45 teeth ring (Autodesk Fusion 360 design; units mm, degrees)
description: Spur Gear; Module: 1.27; Num Teeth: 45; Pressure Angle: 20.0; Backlash: 0.00 mm
part number: 2026-06-12-01-57-33-640
Autodesk Fusion 360 part; units mm, degrees
(part 1 of 5)
sketch "Base Circle" plane through (0, 0, 0) normal (0, 0, 1) x (1, 0, 0)
  circle A0 centre (0, 0) radius 27.1056
  circle A1 centre (0, 0) radius 2.5
extrude "Extrude1" add sketch "Base Circle" along normal blind 1 makes body 1
sketch "Gear Tooth" plane through (0, 0, 0) normal (0, 0, 1) x (1, 0, 0)
  spline S0 degree 5 poles (26.8184, -1.337) (26.8271, -1.337) (26.8445, -1.337) (26.8706, -1.3368) (26.9054, -1.3362) (26.9489, -1.3346) (26.9925, -1.3324) (27.036, -1.3295) (27.0796, -1.3259) (27.1232, -1.3218) (27.1667, -1.3171) (27.2103, -1.3119) (27.2539, -1.3063) (27.2974, -1.3003) (27.341, -1.294) (27.3845, -1.2874) (27.4281, -1.2804) (27.4716, -1.273) (27.5152, -1.2653) (27.5587, -1.2573) (27.6022, -1.249) (27.6457, -1.2403) (27.6892, -1.2313) (27.7327, -1.2221) (27.7762, -1.2126) (27.8196, -1.2028) (27.8631, -1.1927) (27.9065, -1.1824) (27.9499, -1.1718) (27.9933, -1.1609) (28.0367, -1.1498) (28.0801, -1.1384) (28.1235, -1.1268) (28.1668, -1.115) (28.2101, -1.1029) (28.2534, -1.0905) (28.2967, -1.0779) (28.34, -1.0651) (28.3833, -1.0521) (28.4265, -1.0389) (28.4697, -1.0254) (28.513, -1.0117) (28.5561, -0.9978) (28.5993, -0.9837) (28.6424, -0.9693) (28.6856, -0.9548) (28.7287, -0.94) (28.7718, -0.925) (28.8148, -0.9099) (28.8579, -0.8945) (28.9009, -0.8789) (28.9439, -0.8631) (28.9868, -0.8471) (29.0298, -0.831) (29.0727, -0.8146) (29.1156, -0.798) (29.1585, -0.7813) (29.2013, -0.7643) (29.2442, -0.7472) (29.287, -0.7299) (29.3298, -0.7124) (29.3725, -0.6947) (29.4152, -0.6768) (29.4579, -0.6588) (29.5006, -0.6405) (29.5433, -0.6221) (29.5859, -0.6035) (29.6285, -0.5847) (29.671, -0.5658) (29.7136, -0.5466) (29.7561, -0.5273) (29.7901, -0.5118) (29.8155, -0.5) (29.8325, -0.4921) (29.841, -0.4882) knots 0 0 0 0 0 0 0.01428571 0.02857143 0.04285714 0.05714286 0.07142857 0.08571429 0.1 0.11428571 0.12857143 0.14285714 0.15714286 0.17142857 0.18571429 0.2 0.21428571 0.22857143 0.24285714 0.25714286 0.27142857 0.28571429 0.3 0.31428571 0.32857143 0.34285714 0.35714286 0.37142857 0.38571429 0.4 0.41428571 0.42857143 0.44285714 0.45714286 0.47142857 0.48571429 0.5 0.51428571 0.52857143 0.54285714 0.55714286 0.57142857 0.58571429 0.6 0.61428571 0.62857143 0.64285714 0.65714286 0.67142857 0.68571429 0.7 0.71428571 0.72857143 0.74285714 0.75714286 0.77142857 0.78571429 0.8 0.81428571 0.82857143 0.84285714 0.85714286 0.87142857 0.88571429 0.9 0.91428571 0.92857143 0.94285714 0.95714286 0.97142857 0.98571429 1 1 1 1 1 1
  spline S1 degree 5 poles (26.8184, 1.337) (26.8271, 1.337) (26.8445, 1.337) (26.8706, 1.3368) (26.9054, 1.3362) (26.9489, 1.3346) (26.9925, 1.3324) (27.036, 1.3295) (27.0796, 1.3259) (27.1232, 1.3218) (27.1667, 1.3171) (27.2103, 1.3119) (27.2539, 1.3063) (27.2974, 1.3003) (27.341, 1.294) (27.3845, 1.2874) (27.4281, 1.2804) (27.4716, 1.273) (27.5152, 1.2653) (27.5587, 1.2573) (27.6022, 1.249) (27.6457, 1.2403) (27.6892, 1.2313) (27.7327, 1.2221) (27.7762, 1.2126) (27.8196, 1.2028) (27.8631, 1.1927) (27.9065, 1.1824) (27.9499, 1.1718) (27.9933, 1.1609) (28.0367, 1.1498) (28.0801, 1.1384) (28.1235, 1.1268) (28.1668, 1.115) (28.2101, 1.1029) (28.2534, 1.0905) (28.2967, 1.0779) (28.34, 1.0651) (28.3833, 1.0521) (28.4265, 1.0389) (28.4697, 1.0254) (28.513, 1.0117) (28.5561, 0.9978) (28.5993, 0.9837) (28.6424, 0.9693) (28.6856, 0.9548) (28.7287, 0.94) (28.7718, 0.925) (28.8148, 0.9099) (28.8579, 0.8945) (28.9009, 0.8789) (28.9439, 0.8631) (28.9868, 0.8471) (29.0298, 0.831) (29.0727, 0.8146) (29.1156, 0.798) (29.1585, 0.7813) (29.2013, 0.7643) (29.2442, 0.7472) (29.287, 0.7299) (29.3298, 0.7124) (29.3725, 0.6947) (29.4152, 0.6768) (29.4579, 0.6588) (29.5006, 0.6405) (29.5433, 0.6221) (29.5859, 0.6035) (29.6285, 0.5847) (29.671, 0.5658) (29.7136, 0.5466) (29.7561, 0.5273) (29.7901, 0.5118) (29.8155, 0.5) (29.8325, 0.4921) (29.841, 0.4882) knots 0 0 0 0 0 0 0.01428571 0.02857143 0.04285714 0.05714286 0.07142857 0.08571429 0.1 0.11428571 0.12857143 0.14285714 0.15714286 0.17142857 0.18571429 0.2 0.21428571 0.22857143 0.24285714 0.25714286 0.27142857 0.28571429 0.3 0.31428571 0.32857143 0.34285714 0.35714286 0.37142857 0.38571429 0.4 0.41428571 0.42857143 0.44285714 0.45714286 0.47142857 0.48571429 0.5 0.51428571 0.52857143 0.54285714 0.55714286 0.57142857 0.58571429 0.6 0.61428571 0.62857143 0.64285714 0.65714286 0.67142857 0.68571429 0.7 0.71428571 0.72857143 0.74285714 0.75714286 0.77142857 0.78571429 0.8 0.81428571 0.82857143 0.84285714 0.85714286 0.87142857 0.88571429 0.9 0.91428571 0.92857143 0.94285714 0.95714286 0.97142857 0.98571429 1 1 1 1 1 1
  arc A0 (29.841, -0.4882) -> (29.841, 0.4882) centre (0, 0) ccw
  line L0 (26.8184, 1.337) -> (26.8184, -1.337)
  point P0 (27.0328, -1.3296)
  point P1 (27.248, -1.307)
  point P2 (27.4636, -1.2743)
  point P3 (27.6795, -1.2333)
  point P4 (27.8956, -1.1849)
  point P5 (28.1119, -1.1299)
  point P6 (28.3282, -1.0686)
  point P7 (28.5446, -1.0015)
  point P8 (28.761, -0.9287)
  point P9 (28.9773, -0.8507)
  point P10 (29.1935, -0.7674)
  point P11 (29.4095, -0.6792)
  point P12 (29.6254, -0.586)
  point P13 (27.0328, 1.3296)
  point P14 (27.248, 1.307)
  point P15 (27.4636, 1.2743)
  point P16 (27.6795, 1.2333)
  point P17 (27.8956, 1.1849)
  point P18 (28.1119, 1.1299)
  point P19 (28.3282, 1.0686)
  point P20 (28.5446, 1.0015)
  point P21 (28.761, 0.9287)
  point P22 (28.9773, 0.8507)
  point P23 (29.1935, 0.7674)
  point P24 (29.4095, 0.6792)
  point P25 (29.6254, 0.586)
extrude "Extrude2" add sketch "Gear Tooth" along normal blind 1 bodies 1
fillet "Fillet1" radius 0.2 2 edges at (27.0731, 1.3263, 0.5) (27.0731, -1.3263, 0.5) on bodies 1
pattern_circular "C-Pattern1" count 45 over 360 about axis through (0, 0, 0) along (0, 0, 1) of "Extrude2", "Fillet1"
sketch "Diametrial Pitch Circle" plane through (0, 0, 0) normal (0, 0, 1) x (1, 0, 0)
  circle A0 centre (0, 0) radius 28.575 construction
sketch "Sketch4" plane through (0, 0, 1) normal (0, 0, 1) x (1, 0, 0)
  arc A0 (27.0091, -2.2856) -> (27.0643, -1.4956) centre (0, 0) ccw
  spline S0 degree 3 poles (27.2384, -1.3082) (27.2125, -1.3116) (27.1876, -1.3199) (27.1423, -1.3457) (27.1225, -1.3629) (27.0939, -1.3995) (27.0839, -1.4173) (27.0696, -1.4553) (27.0654, -1.4753) (27.0643, -1.4956) knots 0 0 0 0 0.007813 0.007813 0.015626 0.015626 0.021719 0.021719 0.027811 0.027811 0.027811 0.027811
  spline S1 degree 5 poles (27.2384, -1.3082) (27.2415, -1.3078) (27.2533, -1.3063) (27.2738, -1.3036) (27.303, -1.2995) (27.341, -1.294) (27.3845, -1.2874) (27.4281, -1.2804) (27.4716, -1.273) (27.5152, -1.2653) (27.5587, -1.2573) (27.6022, -1.249) (27.6457, -1.2403) (27.6892, -1.2313) (27.7327, -1.2221) (27.7762, -1.2126) (27.8196, -1.2028) (27.8631, -1.1927) (27.9065, -1.1824) (27.9499, -1.1718) (27.9933, -1.1609) (28.0367, -1.1498) (28.0801, -1.1384) (28.1235, -1.1268) (28.1668, -1.115) (28.2101, -1.1029) (28.2534, -1.0905) (28.2967, -1.0779) (28.34, -1.0651) (28.3833, -1.0521) (28.4265, -1.0389) (28.4697, -1.0254) (28.513, -1.0117) (28.5561, -0.9978) (28.5993, -0.9837) (28.6424, -0.9693) (28.6856, -0.9548) (28.7287, -0.94) (28.7718, -0.925) (28.8148, -0.9099) (28.8579, -0.8945) (28.9009, -0.8789) (28.9439, -0.8631) (28.9868, -0.8471) (29.0298, -0.831) (29.0727, -0.8146) (29.1156, -0.798) (29.1585, -0.7813) (29.2013, -0.7643) (29.2442, -0.7472) (29.287, -0.7299) (29.3298, -0.7124) (29.3725, -0.6947) (29.4152, -0.6768) (29.4579, -0.6588) (29.5006, -0.6405) (29.5433, -0.6221) (29.5859, -0.6035) (29.6285, -0.5847) (29.671, -0.5658) (29.7136, -0.5466) (29.7561, -0.5273) (29.7901, -0.5118) (29.8155, -0.5) (29.8325, -0.4921) (29.841, -0.4882) knots 0.13777296 0.13777296 0.13777296 0.13777296 0.13777296 0.13777296 0.14285714 0.15714286 0.17142857 0.18571429 0.2 0.21428571 0.22857143 0.24285714 0.25714286 0.27142857 0.28571429 0.3 0.31428571 0.32857143 0.34285714 0.35714286 0.37142857 0.38571429 0.4 0.41428571 0.42857143 0.44285714 0.45714286 0.47142857 0.48571429 0.5 0.51428571 0.52857143 0.54285714 0.55714286 0.57142857 0.58571429 0.6 0.61428571 0.62857143 0.64285714 0.65714286 0.67142857 0.68571429 0.7 0.71428571 0.72857143 0.74285714 0.75714286 0.77142857 0.78571429 0.8 0.81428571 0.82857143 0.84285714 0.85714286 0.87142857 0.88571429 0.9 0.91428571 0.92857143 0.94285714 0.95714286 0.97142857 0.98571429 1 1 1 1 1 1
  arc A1 (29.841, -0.4882) -> (29.841, 0.4882) centre (0, 0) ccw
  spline S2 degree 5 poles (29.841, 0.4882) (29.8325, 0.4921) (29.8155, 0.5) (29.7901, 0.5118) (29.7561, 0.5273) (29.7136, 0.5466) (29.671, 0.5658) (29.6285, 0.5847) (29.5859, 0.6035) (29.5433, 0.6221) (29.5006, 0.6405) (29.4579, 0.6588) (29.4152, 0.6768) (29.3725, 0.6947) (29.3298, 0.7124) (29.287, 0.7299) (29.2442, 0.7472) (29.2013, 0.7643) (29.1585, 0.7813) (29.1156, 0.798) (29.0727, 0.8146) (29.0298, 0.831) (28.9868, 0.8471) (28.9439, 0.8631) (28.9009, 0.8789) (28.8579, 0.8945) (28.8148, 0.9099) (28.7718, 0.925) (28.7287, 0.94) (28.6856, 0.9548) (28.6424, 0.9693) (28.5993, 0.9837) (28.5561, 0.9978) (28.513, 1.0117) (28.4697, 1.0254) (28.4265, 1.0389) (28.3833, 1.0521) (28.34, 1.0651) (28.2967, 1.0779) (28.2534, 1.0905) (28.2101, 1.1029) (28.1668, 1.115) (28.1235, 1.1268) (28.0801, 1.1384) (28.0367, 1.1498) (27.9933, 1.1609) (27.9499, 1.1718) (27.9065, 1.1824) (27.8631, 1.1927) (27.8196, 1.2028) (27.7762, 1.2126) (27.7327, 1.2221) (27.6892, 1.2313) (27.6457, 1.2403) (27.6022, 1.249) (27.5587, 1.2573) (27.5152, 1.2653) (27.4716, 1.273) (27.4281, 1.2804) (27.3845, 1.2874) (27.341, 1.294) (27.303, 1.2995) (27.2738, 1.3036) (27.2533, 1.3063) (27.2415, 1.3078) (27.2384, 1.3082) knots -1 -1 -1 -1 -1 -1 -0.98571429 -0.97142857 -0.95714286 -0.94285714 -0.92857143 -0.91428571 -0.9 -0.88571429 -0.87142857 -0.85714286 -0.84285714 -0.82857143 -0.81428571 -0.8 -0.78571429 -0.77142857 -0.75714286 -0.74285714 -0.72857143 -0.71428571 -0.7 -0.68571429 -0.67142857 -0.65714286 -0.64285714 -0.62857143 -0.61428571 -0.6 -0.58571429 -0.57142857 -0.55714286 -0.54285714 -0.52857143 -0.51428571 -0.5 -0.48571429 -0.47142857 -0.45714286 -0.44285714 -0.42857143 -0.41428571 -0.4 -0.38571429 -0.37142857 -0.35714286 -0.34285714 -0.32857143 -0.31428571 -0.3 -0.28571429 -0.27142857 -0.25714286 -0.24285714 -0.22857143 -0.21428571 -0.2 -0.18571429 -0.17142857 -0.15714286 -0.14285714 -0.13777296 -0.13777296 -0.13777296 -0.13777296 -0.13777296 -0.13777296
  spline S3 degree 3 poles (27.0643, 1.4956) (27.0658, 1.4696) (27.0723, 1.4441) (27.0947, 1.3971) (27.1103, 1.376) (27.1447, 1.3448) (27.1617, 1.3335) (27.1986, 1.3165) (27.2182, 1.3109) (27.2384, 1.3082) knots 0 0 0 0 0.007813 0.007813 0.015626 0.015626 0.021719 0.021719 0.027811 0.027811 0.027811 0.027811
  arc A2 (27.0643, 1.4956) -> (27.0091, 2.2856) centre (0, 0) ccw
  spline S4 degree 3 poles (27.1553, 2.4953) (27.1302, 2.4884) (27.1067, 2.4767) (27.0655, 2.4448) (27.0482, 2.4251) (27.025, 2.3849) (27.0176, 2.3659) (27.0087, 2.3262) (27.0074, 2.3059) (27.0091, 2.2856) knots 0 0 0 0 0.007813 0.007813 0.015626 0.015626 0.021719 0.021719 0.027811 0.027811 0.027811 0.027811
  spline S5 degree 5 poles (27.1553, 2.4953) (27.1584, 2.4962) (27.1698, 2.4993) (27.1898, 2.5049) (27.2182, 2.513) (27.255, 2.5237) (27.2972, 2.5364) (27.3393, 2.5493) (27.3814, 2.5627) (27.4235, 2.5764) (27.4655, 2.5904) (27.5074, 2.6047) (27.5493, 2.6193) (27.5911, 2.6342) (27.6329, 2.6494) (27.6746, 2.6649) (27.7163, 2.6807) (27.7579, 2.6967) (27.7995, 2.713) (27.841, 2.7295) (27.8825, 2.7463) (27.9239, 2.7633) (27.9653, 2.7806) (28.0066, 2.7982) (28.0479, 2.816) (28.0891, 2.834) (28.1303, 2.8522) (28.1714, 2.8707) (28.2125, 2.8894) (28.2535, 2.9083) (28.2945, 2.9275) (28.3354, 2.9468) (28.3763, 2.9664) (28.4171, 2.9862) (28.4579, 3.0062) (28.4986, 3.0264) (28.5393, 3.0468) (28.5799, 3.0674) (28.6205, 3.0882) (28.661, 3.1092) (28.7015, 3.1305) (28.7419, 3.1519) (28.7823, 3.1735) (28.8226, 3.1953) (28.8629, 3.2173) (28.9032, 3.2395) (28.9433, 3.2618) (28.9835, 3.2844) (29.0235, 3.3071) (29.0636, 3.3301) (29.1035, 3.3532) (29.1435, 3.3765) (29.1833, 3.3999) (29.2232, 3.4236) (29.2629, 3.4474) (29.3027, 3.4714) (29.3423, 3.4956) (29.3819, 3.5199) (29.4215, 3.5445) (29.461, 3.5691) (29.5005, 3.594) (29.5399, 3.619) (29.5714, 3.6392) (29.595, 3.6544) (29.6107, 3.6646) (29.6185, 3.6697) knots 0.13777296 0.13777296 0.13777296 0.13777296 0.13777296 0.13777296 0.14285714 0.15714286 0.17142857 0.18571429 0.2 0.21428571 0.22857143 0.24285714 0.25714286 0.27142857 0.28571429 0.3 0.31428571 0.32857143 0.34285714 0.35714286 0.37142857 0.38571429 0.4 0.41428571 0.42857143 0.44285714 0.45714286 0.47142857 0.48571429 0.5 0.51428571 0.52857143 0.54285714 0.55714286 0.57142857 0.58571429 0.6 0.61428571 0.62857143 0.64285714 0.65714286 0.67142857 0.68571429 0.7 0.71428571 0.72857143 0.74285714 0.75714286 0.77142857 0.78571429 0.8 0.81428571 0.82857143 0.84285714 0.85714286 0.87142857 0.88571429 0.9 0.91428571 0.92857143 0.94285714 0.95714286 0.97142857 0.98571429 1 1 1 1 1 1
  arc A3 (29.6185, 3.6697) -> (29.4827, 4.6365) centre (0, 0) ccw
  spline S6 degree 5 poles (29.4827, 4.6365) (29.4737, 4.6392) (29.4558, 4.6446) (29.4289, 4.6527) (29.3931, 4.6634) (29.3483, 4.6766) (29.3035, 4.6897) (29.2588, 4.7025) (29.214, 4.7152) (29.1692, 4.7277) (29.1244, 4.74) (29.0796, 4.7521) (29.0348, 4.764) (28.99, 4.7758) (28.9452, 4.7874) (28.9004, 4.7987) (28.8556, 4.8099) (28.8108, 4.8209) (28.766, 4.8318) (28.7212, 4.8424) (28.6764, 4.8528) (28.6316, 4.863) (28.5868, 4.8731) (28.5421, 4.8829) (28.4973, 4.8926) (28.4525, 4.902) (28.4078, 4.9112) (28.363, 4.9203) (28.3183, 4.9291) (28.2735, 4.9377) (28.2288, 4.9461) (28.1841, 4.9543) (28.1394, 4.9623) (28.0947, 4.9701) (28.05, 4.9776) (28.0053, 4.985) (27.9606, 4.9921) (27.916, 4.999) (27.8713, 5.0056) (27.8267, 5.012) (27.7821, 5.0182) (27.7375, 5.0242) (27.6929, 5.0299) (27.6484, 5.0353) (27.6038, 5.0406) (27.5593, 5.0455) (27.5148, 5.0503) (27.4704, 5.0547) (27.4259, 5.0589) (27.3815, 5.0628) (27.3371, 5.0665) (27.2927, 5.0699) (27.2484, 5.073) (27.204, 5.0758) (27.1598, 5.0783) (27.1155, 5.0805) (27.0713, 5.0824) (27.0271, 5.0839) (26.983, 5.0852) (26.9389, 5.086) (26.8948, 5.0866) (26.8565, 5.0867) (26.827, 5.0867) (26.8062, 5.0865) (26.7943, 5.0864) (26.7912, 5.0864) knots -1 -1 -1 -1 -1 -1 -0.98571429 -0.97142857 -0.95714286 -0.94285714 -0.92857143 -0.91428571 -0.9 -0.88571429 -0.87142857 -0.85714286 -0.84285714 -0.82857143 -0.81428571 -0.8 -0.78571429 -0.77142857 -0.75714286 -0.74285714 -0.72857143 -0.71428571 -0.7 -0.68571429 -0.67142857 -0.65714286 -0.64285714 -0.62857143 -0.61428571 -0.6 -0.58571429 -0.57142857 -0.55714286 -0.54285714 -0.52857143 -0.51428571 -0.5 -0.48571429 -0.47142857 -0.45714286 -0.44285714 -0.42857143 -0.41428571 -0.4 -0.38571429 -0.37142857 -0.35714286 -0.34285714 -0.32857143 -0.31428571 -0.3 -0.28571429 -0.27142857 -0.25714286 -0.24285714 -0.22857143 -0.21428571 -0.2 -0.18571429 -0.17142857 -0.15714286 -0.14285714 -0.13777296 -0.13777296 -0.13777296 -0.13777296 -0.13777296 -0.13777296
  spline S7 degree 3 poles (26.5928, 5.2476) (26.5978, 5.2221) (26.6078, 5.1978) (26.6365, 5.1543) (26.655, 5.1356) (26.6933, 5.1095) (26.7118, 5.1007) (26.7507, 5.089) (26.7709, 5.0861) (26.7912, 5.0864) knots 0 0 0 0 0.007813 0.007813 0.015626 0.015626 0.021719 0.021719 0.027811 0.027811 0.027811 0.027811
  arc A4 (26.5928, 5.2476) -> (26.4281, 6.0223) centre (0, 0) ccw
  spline S8 degree 3 poles (26.5438, 6.2503) (26.5199, 6.24) (26.4982, 6.2251) (26.4618, 6.1878) (26.4475, 6.1658) (26.4301, 6.1229) (26.4254, 6.103) (26.4221, 6.0625) (26.4236, 6.0421) (26.4281, 6.0223) knots 0 0 0 0 0.007813 0.007813 0.015626 0.015626 0.021719 0.021719 0.027811 0.027811 0.027811 0.027811
  spline S9 degree 5 poles (26.5438, 6.2503) (26.5467, 6.2516) (26.5576, 6.2563) (26.5766, 6.2646) (26.6036, 6.2765) (26.6385, 6.2923) (26.6786, 6.3107) (26.7185, 6.3294) (26.7583, 6.3485) (26.798, 6.3679) (26.8377, 6.3876) (26.8772, 6.4076) (26.9166, 6.4279) (26.956, 6.4485) (26.9952, 6.4694) (27.0344, 6.4905) (27.0735, 6.5119) (27.1125, 6.5336) (27.1514, 6.5555) (27.1902, 6.5777) (27.2289, 6.6001) (27.2676, 6.6227) (27.3061, 6.6456) (27.3446, 6.6687) (27.383, 6.6921) (27.4213, 6.7156) (27.4595, 6.7394) (27.4977, 6.7634) (27.5358, 6.7877) (27.5738, 6.8121) (27.6117, 6.8368) (27.6495, 6.8617) (27.6873, 6.8867) (27.7249, 6.912) (27.7625, 6.9375) (27.8001, 6.9632) (27.8375, 6.989) (27.8749, 7.0151) (27.9122, 7.0414) (27.9494, 7.0678) (27.9865, 7.0945) (28.0236, 7.1213) (28.0605, 7.1483) (28.0974, 7.1755) (28.1343, 7.2029) (28.171, 7.2305) (28.2077, 7.2582) (28.2443, 7.2861) (28.2808, 7.3142) (28.3173, 7.3425) (28.3536, 7.371) (28.3899, 7.3996) (28.4262, 7.4284) (28.4623, 7.4573) (28.4984, 7.4865) (28.5344, 7.5158) (28.5703, 7.5452) (28.6061, 7.5749) (28.6419, 7.6046) (28.6776, 7.6346) (28.7132, 7.6647) (28.7487, 7.695) (28.7771, 7.7193) (28.7984, 7.7377) (28.8125, 7.7499) (28.8196, 7.756) knots 0.13777296 0.13777296 0.13777296 0.13777296 0.13777296 0.13777296 0.14285714 0.15714286 0.17142857 0.18571429 0.2 0.21428571 0.22857143 0.24285714 0.25714286 0.27142857 0.28571429 0.3 0.31428571 0.32857143 0.34285714 0.35714286 0.37142857 0.38571429 0.4 0.41428571 0.42857143 0.44285714 0.45714286 0.47142857 0.48571429 0.5 0.51428571 0.52857143 0.54285714 0.55714286 0.57142857 0.58571429 0.6 0.61428571 0.62857143 0.64285714 0.65714286 0.67142857 0.68571429 0.7 0.71428571 0.72857143 0.74285714 0.75714286 0.77142857 0.78571429 0.8 0.81428571 0.82857143 0.84285714 0.85714286 0.87142857 0.88571429 0.9 0.91428571 0.92857143 0.94285714 0.95714286 0.97142857 0.98571429 1 1 1 1 1 1
  arc A5 (28.8196, 7.756) -> (28.5505, 8.6945) centre (0, 0) ccw
  spline S10 degree 5 poles (28.5505, 8.6945) (28.5412, 8.696) (28.5227, 8.6989) (28.495, 8.7032) (28.458, 8.7088) (28.4118, 8.7156) (28.3657, 8.7223) (28.3195, 8.7288) (28.2734, 8.7351) (28.2273, 8.7412) (28.1813, 8.7472) (28.1352, 8.7529) (28.0892, 8.7585) (28.0432, 8.7639) (27.9972, 8.7692) (27.9513, 8.7742) (27.9053, 8.7791) (27.8595, 8.7837) (27.8136, 8.7882) (27.7678, 8.7925) (27.722, 8.7966) (27.6762, 8.8005) (27.6304, 8.8042) (27.5847, 8.8077) (27.539, 8.811) (27.4934, 8.8141) (27.4478, 8.817) (27.4022, 8.8198) (27.3567, 8.8223) (27.3112, 8.8246) (27.2657, 8.8267) (27.2203, 8.8286) (27.1749, 8.8303) (27.1295, 8.8317) (27.0842, 8.833) (27.039, 8.834) (26.9938, 8.8349) (26.9486, 8.8355) (26.9035, 8.8358) (26.8584, 8.836) (26.8133, 8.8359) (26.7683, 8.8356) (26.7234, 8.835) (26.6785, 8.8343) (26.6337, 8.8332) (26.5889, 8.832) (26.5442, 8.8304) (26.4995, 8.8287) (26.4549, 8.8266) (26.4104, 8.8243) (26.3659, 8.8218) (26.3215, 8.8189) (26.2772, 8.8158) (26.2329, 8.8124) (26.1887, 8.8088) (26.1445, 8.8048) (26.1005, 8.8005) (26.0565, 8.7959) (26.0127, 8.791) (25.9689, 8.7857) (25.9252, 8.7801) (25.8872, 8.7749) (25.8579, 8.7708) (25.8375, 8.7677) (25.8257, 8.7659) (25.8226, 8.7655) knots -1 -1 -1 -1 -1 -1 -0.98571429 -0.97142857 -0.95714286 -0.94285714 -0.92857143 -0.91428571 -0.9 -0.88571429 -0.87142857 -0.85714286 -0.84285714 -0.82857143 -0.81428571 -0.8 -0.78571429 -0.77142857 -0.75714286 -0.74285714 -0.72857143 -0.71428571 -0.7 -0.68571429 -0.67142857 -0.65714286 -0.64285714 -0.62857143 -0.61428571 -0.6 -0.58571429 -0.57142857 -0.55714286 -0.54285714 -0.52857143 -0.51428571 -0.5 -0.48571429 -0.47142857 -0.45714286 -0.44285714 -0.42857143 -0.41428571 -0.4 -0.38571429 -0.37142857 -0.35714286 -0.34285714 -0.32857143 -0.31428571 -0.3 -0.28571429 -0.27142857 -0.25714286 -0.24285714 -0.22857143 -0.21428571 -0.2 -0.18571429 -0.17142857 -0.15714286 -0.14285714 -0.13777296 -0.13777296 -0.13777296 -0.13777296 -0.13777296 -0.13777296
  spline S11 degree 3 poles (25.6037, 8.8976) (25.6122, 8.873) (25.6255, 8.8503) (25.66, 8.8112) (25.6809, 8.7953) (25.7225, 8.7748) (25.7419, 8.7687) (25.7821, 8.7625) (25.8025, 8.7624) (25.8226, 8.7655) knots 0 0 0 0 0.007813 0.007813 0.015626 0.015626 0.021719 0.021719 0.027811 0.027811 0.027811 0.027811
  arc A6 (25.6037, 8.8976) -> (25.3328, 9.6418) centre (0, 0) ccw
  spline S12 degree 3 poles (25.4156, 9.8837) (25.3934, 9.8701) (25.374, 9.8524) (25.3431, 9.8104) (25.332, 9.7866) (25.3207, 9.7416) (25.3188, 9.7213) (25.3213, 9.6807) (25.3256, 9.6608) (25.3328, 9.6418) knots 0 0 0 0 0.007813 0.007813 0.015626 0.015626 0.021719 0.021719 0.027811 0.027811 0.027811 0.027811
  spline S13 degree 5 poles (25.4156, 9.8837) (25.4183, 9.8853) (25.4284, 9.8915) (25.4461, 9.9024) (25.4711, 9.918) (25.5036, 9.9384) (25.5406, 9.9622) (25.5776, 9.9863) (25.6144, 10.0108) (25.651, 10.0355) (25.6875, 10.0605) (25.7239, 10.0858) (25.7601, 10.1114) (25.7962, 10.1373) (25.8321, 10.1634) (25.868, 10.1898) (25.9037, 10.2165) (25.9393, 10.2433) (25.9748, 10.2704) (26.0101, 10.2978) (26.0454, 10.3254) (26.0805, 10.3532) (26.1155, 10.3812) (26.1504, 10.4094) (26.1851, 10.4379) (26.2198, 10.4666) (26.2544, 10.4955) (26.2888, 10.5246) (26.3231, 10.5539) (26.3574, 10.5834) (26.3915, 10.6131) (26.4255, 10.6429) (26.4594, 10.673) (26.4932, 10.7033) (26.5268, 10.7338) (26.5604, 10.7644) (26.5939, 10.7953) (26.6273, 10.8263) (26.6606, 10.8575) (26.6937, 10.8889) (26.7268, 10.9204) (26.7597, 10.9521) (26.7926, 10.984) (26.8254, 11.0161) (26.858, 11.0484) (26.8906, 11.0808) (26.923, 11.1133) (26.9554, 11.1461) (26.9876, 11.179) (27.0198, 11.2121) (27.0519, 11.2453) (27.0838, 11.2787) (27.1157, 11.3122) (27.1474, 11.346) (27.1791, 11.3798) (27.2107, 11.4138) (27.2421, 11.448) (27.2735, 11.4823) (27.3048, 11.5168) (27.336, 11.5514) (27.367, 11.5862) (27.398, 11.6211) (27.4227, 11.6492) (27.4412, 11.6703) (27.4535, 11.6844) (27.4597, 11.6915) knots 0.13777296 0.13777296 0.13777296 0.13777296 0.13777296 0.13777296 0.14285714 0.15714286 0.17142857 0.18571429 0.2 0.21428571 0.22857143 0.24285714 0.25714286 0.27142857 0.28571429 0.3 0.31428571 0.32857143 0.34285714 0.35714286 0.37142857 0.38571429 0.4 0.41428571 0.42857143 0.44285714 0.45714286 0.47142857 0.48571429 0.5 0.51428571 0.52857143 0.54285714 0.55714286 0.57142857 0.58571429 0.6 0.61428571 0.62857143 0.64285714 0.65714286 0.67142857 0.68571429 0.7 0.71428571 0.72857143 0.74285714 0.75714286 0.77142857 0.78571429 0.8 0.81428571 0.82857143 0.84285714 0.85714286 0.87142857 0.88571429 0.9 0.91428571 0.92857143 0.94285714 0.95714286 0.97142857 0.98571429 1 1 1 1 1 1
  arc A7 (27.4597, 11.6915) -> (27.0626, 12.5834) centre (0, 0) ccw
  spline S14 degree 5 poles (27.0626, 12.5834) (27.0532, 12.5835) (27.0345, 12.5838) (27.0064, 12.5842) (26.969, 12.5846) (26.9224, 12.585) (26.8757, 12.5852) (26.8291, 12.5852) (26.7826, 12.585) (26.7361, 12.5846) (26.6896, 12.5841) (26.6432, 12.5834) (26.5969, 12.5826) (26.5506, 12.5815) (26.5043, 12.5803) (26.4581, 12.5789) (26.412, 12.5773) (26.3659, 12.5755) (26.3198, 12.5736) (26.2738, 12.5714) (26.2279, 12.5691) (26.182, 12.5666) (26.1362, 12.5639) (26.0905, 12.561) (26.0448, 12.558) (25.9991, 12.5547) (25.9536, 12.5512) (25.9081, 12.5476) (25.8626, 12.5437) (25.8172, 12.5397) (25.7719, 12.5354) (25.7267, 12.531) (25.6815, 12.5263) (25.6364, 12.5215) (25.5913, 12.5164) (25.5464, 12.5112) (25.5015, 12.5057) (25.4567, 12.5) (25.4119, 12.4941) (25.3673, 12.4879) (25.3227, 12.4816) (25.2782, 12.475) (25.2337, 12.4682) (25.1894, 12.4612) (25.1452, 12.454) (25.101, 12.4465) (25.0569, 12.4387) (25.0129, 12.4308) (24.9691, 12.4225) (24.9253, 12.4141) (24.8816, 12.4053) (24.838, 12.3963) (24.7945, 12.3871) (24.7511, 12.3776) (24.7079, 12.3678) (24.6647, 12.3577) (24.6217, 12.3474) (24.5788, 12.3367) (24.536, 12.3257) (24.4934, 12.3144) (24.4509, 12.3027) (24.414, 12.2923) (24.3856, 12.2841) (24.3658, 12.2783) (24.3544, 12.2749) (24.3514, 12.274) knots -1 -1 -1 -1 -1 -1 -0.98571429 -0.97142857 -0.95714286 -0.94285714 -0.92857143 -0.91428571 -0.9 -0.88571429 -0.87142857 -0.85714286 -0.84285714 -0.82857143 -0.81428571 -0.8 -0.78571429 -0.77142857 -0.75714286 -0.74285714 -0.72857143 -0.71428571 -0.7 -0.68571429 -0.67142857 -0.65714286 -0.64285714 -0.62857143 -0.61428571 -0.6 -0.58571429 -0.57142857 -0.55714286 -0.54285714 -0.52857143 -0.51428571 -0.5 -0.48571429 -0.47142857 -0.45714286 -0.44285714 -0.42857143 -0.41428571 -0.4 -0.38571429 -0.37142857 -0.35714286 -0.34285714 -0.32857143 -0.31428571 -0.3 -0.28571429 -0.27142857 -0.25714286 -0.24285714 -0.22857143 -0.21428571 -0.2 -0.18571429 -0.17142857 -0.15714286 -0.14285714 -0.13777296 -0.13777296 -0.13777296 -0.13777296 -0.13777296 -0.13777296
  spline S15 degree 3 poles (24.1162, 12.3743) (24.1281, 12.3511) (24.1444, 12.3305) (24.184, 12.2967) (24.2069, 12.2838) (24.2509, 12.2693) (24.2711, 12.2659) (24.3117, 12.2654) (24.3319, 12.2682) (24.3514, 12.274) knots 0 0 0 0 0.007813 0.007813 0.015626 0.015626 0.021719 0.021719 0.027811 0.027811 0.027811 0.027811
  arc A8 (24.1162, 12.3743) -> (23.7444, 13.0736) centre (0, 0) ccw
  spline S16 degree 3 poles (23.7927, 13.3247) (23.7726, 13.3082) (23.7559, 13.2879) (23.7311, 13.242) (23.7234, 13.2169) (23.7185, 13.1708) (23.7195, 13.1504) (23.7275, 13.1106) (23.7346, 13.0914) (23.7444, 13.0736) knots 0 0 0 0 0.007813 0.007813 0.015626 0.015626 0.021719 0.021719 0.027811 0.027811 0.027811 0.027811
  spline S17 degree 5 poles (23.7927, 13.3247) (23.7951, 13.3267) (23.8043, 13.3342) (23.8203, 13.3474) (23.8429, 13.3663) (23.8722, 13.3911) (23.9056, 13.4198) (23.9388, 13.4489) (23.9719, 13.4782) (24.0047, 13.5077) (24.0374, 13.5376) (24.0698, 13.5678) (24.1021, 13.5982) (24.1343, 13.6288) (24.1663, 13.6597) (24.1981, 13.6908) (24.2298, 13.7221) (24.2613, 13.7537) (24.2926, 13.7855) (24.3238, 13.8175) (24.3549, 13.8497) (24.3858, 13.8821) (24.4165, 13.9147) (24.4472, 13.9476) (24.4776, 13.9806) (24.508, 14.0138) (24.5382, 14.0472) (24.5682, 14.0808) (24.5981, 14.1146) (24.6279, 14.1486) (24.6576, 14.1828) (24.6871, 14.2171) (24.7165, 14.2516) (24.7457, 14.2863) (24.7748, 14.3211) (24.8038, 14.3562) (24.8327, 14.3914) (24.8614, 14.4267) (24.89, 14.4622) (24.9185, 14.4979) (24.9469, 14.5338) (24.9751, 14.5698) (25.0032, 14.6059) (25.0312, 14.6423) (25.059, 14.6787) (25.0867, 14.7154) (25.1143, 14.7522) (25.1418, 14.7891) (25.1692, 14.8262) (25.1964, 14.8634) (25.2236, 14.9008) (25.2506, 14.9383) (25.2774, 14.9759) (25.3042, 15.0137) (25.3308, 15.0517) (25.3574, 15.0898) (25.3838, 15.128) (25.4101, 15.1663) (25.4362, 15.2048) (25.4623, 15.2435) (25.4882, 15.2822) (25.514, 15.3211) (25.5346, 15.3523) (25.55, 15.3758) (25.5602, 15.3915) (25.5653, 15.3993) knots 0.13777296 0.13777296 0.13777296 0.13777296 0.13777296 0.13777296 0.14285714 0.15714286 0.17142857 0.18571429 0.2 0.21428571 0.22857143 0.24285714 0.25714286 0.27142857 0.28571429 0.3 0.31428571 0.32857143 0.34285714 0.35714286 0.37142857 0.38571429 0.4 0.41428571 0.42857143 0.44285714 0.45714286 0.47142857 0.48571429 0.5 0.51428571 0.52857143 0.54285714 0.55714286 0.57142857 0.58571429 0.6 0.61428571 0.62857143 0.64285714 0.65714286 0.67142857 0.68571429 0.7 0.71428571 0.72857143 0.74285714 0.75714286 0.77142857 0.78571429 0.8 0.81428571 0.82857143 0.84285714 0.85714286 0.87142857 0.88571429 0.9 0.91428571 0.92857143 0.94285714 0.95714286 0.97142857 0.98571429 1 1 1 1 1 1
  arc A9 (25.5653, 15.3993) -> (25.0479, 16.2273) centre (0, 0) ccw
  spline S18 degree 5 poles (25.0479, 16.2273) (25.0386, 16.2262) (25.0201, 16.2238) (24.9922, 16.2203) (24.9551, 16.2155) (24.9089, 16.2094) (24.8627, 16.2031) (24.8165, 16.1966) (24.7704, 16.1899) (24.7244, 16.1831) (24.6785, 16.1761) (24.6327, 16.169) (24.5869, 16.1617) (24.5412, 16.1542) (24.4955, 16.1465) (24.45, 16.1387) (24.4045, 16.1307) (24.3591, 16.1226) (24.3138, 16.1142) (24.2685, 16.1057) (24.2234, 16.097) (24.1783, 16.0881) (24.1333, 16.0791) (24.0884, 16.0699) (24.0436, 16.0605) (23.9989, 16.0509) (23.9542, 16.0411) (23.9096, 16.0312) (23.8652, 16.021) (23.8208, 16.0107) (23.7765, 16.0002) (23.7323, 15.9895) (23.6882, 15.9786) (23.6442, 15.9675) (23.6003, 15.9562) (23.5565, 15.9448) (23.5128, 15.9331) (23.4693, 15.9212) (23.4258, 15.9091) (23.3824, 15.8969) (23.3391, 15.8844) (23.296, 15.8717) (23.2529, 15.8588) (23.21, 15.8456) (23.1672, 15.8323) (23.1245, 15.8187) (23.0819, 15.8049) (23.0395, 15.7909) (22.9972, 15.7767) (22.955, 15.7622) (22.9129, 15.7475) (22.871, 15.7325) (22.8293, 15.7173) (22.7876, 15.7018) (22.7461, 15.6861) (22.7048, 15.6701) (22.6637, 15.6539) (22.6227, 15.6373) (22.5818, 15.6205) (22.5412, 15.6033) (22.5007, 15.5859) (22.4656, 15.5705) (22.4387, 15.5584) (22.4198, 15.5498) (22.409, 15.5449) (22.4062, 15.5436) knots -1 -1 -1 -1 -1 -1 -0.98571429 -0.97142857 -0.95714286 -0.94285714 -0.92857143 -0.91428571 -0.9 -0.88571429 -0.87142857 -0.85714286 -0.84285714 -0.82857143 -0.81428571 -0.8 -0.78571429 -0.77142857 -0.75714286 -0.74285714 -0.72857143 -0.71428571 -0.7 -0.68571429 -0.67142857 -0.65714286 -0.64285714 -0.62857143 -0.61428571 -0.6 -0.58571429 -0.57142857 -0.55714286 -0.54285714 -0.52857143 -0.51428571 -0.5 -0.48571429 -0.47142857 -0.45714286 -0.44285714 -0.42857143 -0.41428571 -0.4 -0.38571429 -0.37142857 -0.35714286 -0.34285714 -0.32857143 -0.31428571 -0.3 -0.28571429 -0.27142857 -0.25714286 -0.24285714 -0.22857143 -0.21428571 -0.2 -0.18571429 -0.17142857 -0.15714286 -0.14285714 -0.13777296 -0.13777296 -0.13777296 -0.13777296 -0.13777296 -0.13777296
  spline S19 degree 3 poles (22.1593, 15.6102) (22.1743, 15.5889) (22.1933, 15.5708) (22.2372, 15.5428) (22.2617, 15.5332) (22.3073, 15.525) (22.3278, 15.5244) (22.3681, 15.5295) (22.3877, 15.5351) (22.4062, 15.5436) knots 0 0 0 0 0.007813 0.007813 0.015626 0.015626 0.021719 0.021719 0.027811 0.027811 0.027811 0.027811
  arc A10 (22.1593, 15.6102) -> (21.6938, 16.2509) centre (0, 0) ccw
  spline S20 degree 3 poles (21.7067, 16.5063) (21.6891, 16.4871) (21.6754, 16.4647) (21.6573, 16.4159) (21.6531, 16.3899) (21.6547, 16.3436) (21.6585, 16.3235) (21.672, 16.2852) (21.6816, 16.2672) (21.6938, 16.2509) knots 0 0 0 0 0.007813 0.007813 0.015626 0.015626 0.021719 0.021719 0.027811 0.027811 0.027811 0.027811
  spline S21 degree 5 poles (21.7067, 16.5063) (21.7088, 16.5086) (21.7169, 16.5174) (21.7309, 16.5327) (21.7507, 16.5546) (21.7762, 16.5832) (21.8053, 16.6163) (21.8341, 16.6496) (21.8628, 16.6832) (21.8912, 16.7171) (21.9194, 16.7512) (21.9473, 16.7856) (21.9751, 16.8202) (22.0027, 16.855) (22.03, 16.89) (22.0572, 16.9253) (22.0842, 16.9607) (22.111, 16.9964) (22.1376, 17.0322) (22.1641, 17.0682) (22.1904, 17.1044) (22.2165, 17.1409) (22.2424, 17.1774) (22.2681, 17.2142) (22.2937, 17.2512) (22.3191, 17.2883) (22.3444, 17.3256) (22.3695, 17.363) (22.3944, 17.4007) (22.4191, 17.4385) (22.4438, 17.4764) (22.4682, 17.5145) (22.4925, 17.5528) (22.5166, 17.5912) (22.5406, 17.6298) (22.5644, 17.6685) (22.5881, 17.7073) (22.6117, 17.7464) (22.635, 17.7855) (22.6583, 17.8248) (22.6814, 17.8643) (22.7043, 17.9039) (22.7271, 17.9436) (22.7497, 17.9834) (22.7722, 18.0234) (22.7946, 18.0636) (22.8168, 18.1038) (22.8389, 18.1442) (22.8608, 18.1847) (22.8826, 18.2254) (22.9043, 18.2662) (22.9258, 18.3071) (22.9472, 18.3481) (22.9684, 18.3893) (22.9895, 18.4306) (23.0105, 18.472) (23.0313, 18.5135) (23.052, 18.5551) (23.0726, 18.5969) (23.093, 18.6388) (23.1133, 18.6808) (23.1334, 18.7229) (23.1495, 18.7567) (23.1614, 18.7821) (23.1694, 18.799) (23.1733, 18.8075) knots 0.13777296 0.13777296 0.13777296 0.13777296 0.13777296 0.13777296 0.14285714 0.15714286 0.17142857 0.18571429 0.2 0.21428571 0.22857143 0.24285714 0.25714286 0.27142857 0.28571429 0.3 0.31428571 0.32857143 0.34285714 0.35714286 0.37142857 0.38571429 0.4 0.41428571 0.42857143 0.44285714 0.45714286 0.47142857 0.48571429 0.5 0.51428571 0.52857143 0.54285714 0.55714286 0.57142857 0.58571429 0.6 0.61428571 0.62857143 0.64285714 0.65714286 0.67142857 0.68571429 0.7 0.71428571 0.72857143 0.74285714 0.75714286 0.77142857 0.78571429 0.8 0.81428571 0.82857143 0.84285714 0.85714286 0.87142857 0.88571429 0.9 0.91428571 0.92857143 0.94285714 0.95714286 0.97142857 0.98571429 1 1 1 1 1 1
  arc A11 (23.1733, 18.8075) -> (22.5458, 19.5554) centre (0, 0) ccw
  spline S22 degree 5 poles (22.5458, 19.5554) (22.5367, 19.5529) (22.5186, 19.5481) (22.4916, 19.5407) (22.4555, 19.5308) (22.4105, 19.5183) (22.3657, 19.5056) (22.3209, 19.4927) (22.2762, 19.4797) (22.2316, 19.4666) (22.1871, 19.4533) (22.1426, 19.4398) (22.0983, 19.4262) (22.0541, 19.4125) (22.01, 19.3985) (21.966, 19.3844) (21.922, 19.3702) (21.8782, 19.3558) (21.8345, 19.3412) (21.7909, 19.3265) (21.7474, 19.3116) (21.704, 19.2965) (21.6607, 19.2813) (21.6175, 19.2659) (21.5744, 19.2504) (21.5314, 19.2347) (21.4886, 19.2188) (21.4458, 19.2027) (21.4032, 19.1865) (21.3607, 19.1701) (21.3183, 19.1535) (21.2761, 19.1368) (21.2339, 19.1199) (21.1919, 19.1028) (21.15, 19.0855) (21.1082, 19.068) (21.0666, 19.0504) (21.0251, 19.0326) (20.9837, 19.0146) (20.9424, 18.9963) (20.9013, 18.978) (20.8603, 18.9594) (20.8195, 18.9406) (20.7788, 18.9216) (20.7383, 18.9025) (20.6979, 18.8831) (20.6577, 18.8635) (20.6176, 18.8437) (20.5777, 18.8237) (20.5379, 18.8035) (20.4983, 18.7831) (20.4589, 18.7624) (20.4197, 18.7415) (20.3806, 18.7204) (20.3417, 18.6991) (20.303, 18.6775) (20.2645, 18.6557) (20.2262, 18.6336) (20.1881, 18.6113) (20.1503, 18.5886) (20.1126, 18.5657) (20.08, 18.5456) (20.055, 18.5299) (20.0375, 18.5188) (20.0275, 18.5123) (20.0249, 18.5107) knots -1 -1 -1 -1 -1 -1 -0.98571429 -0.97142857 -0.95714286 -0.94285714 -0.92857143 -0.91428571 -0.9 -0.88571429 -0.87142857 -0.85714286 -0.84285714 -0.82857143 -0.81428571 -0.8 -0.78571429 -0.77142857 -0.75714286 -0.74285714 -0.72857143 -0.71428571 -0.7 -0.68571429 -0.67142857 -0.65714286 -0.64285714 -0.62857143 -0.61428571 -0.6 -0.58571429 -0.57142857 -0.55714286 -0.54285714 -0.52857143 -0.51428571 -0.5 -0.48571429 -0.47142857 -0.45714286 -0.44285714 -0.42857143 -0.41428571 -0.4 -0.38571429 -0.37142857 -0.35714286 -0.34285714 -0.32857143 -0.31428571 -0.3 -0.28571429 -0.27142857 -0.25714286 -0.24285714 -0.22857143 -0.21428571 -0.2 -0.18571429 -0.17142857 -0.15714286 -0.14285714 -0.13777296 -0.13777296 -0.13777296 -0.13777296 -0.13777296 -0.13777296
  spline S23 degree 3 poles (19.7711, 18.5423) (19.789, 18.5233) (19.8103, 18.5079) (19.8577, 18.4863) (19.8833, 18.4802) (19.9296, 18.4785) (19.9499, 18.4808) (19.9891, 18.4914) (20.0078, 18.4997) (20.0249, 18.5107) knots 0 0 0 0 0.007813 0.007813 0.015626 0.015626 0.021719 0.021719 0.027811 0.027811 0.027811 0.027811
  arc A12 (19.7711, 18.5423) -> (19.221, 19.112) centre (0, 0) ccw
  spline S24 degree 3 poles (19.1982, 19.3667) (19.1834, 19.3452) (19.173, 19.3211) (19.1619, 19.2702) (19.1613, 19.2439) (19.1694, 19.1983) (19.1759, 19.1789) (19.1946, 19.1429) (19.2067, 19.1264) (19.221, 19.112) knots 0 0 0 0 0.007813 0.007813 0.015626 0.015626 0.021719 0.021719 0.027811 0.027811 0.027811 0.027811
  spline S25 degree 5 poles (19.1982, 19.3667) (19.2, 19.3692) (19.2068, 19.379) (19.2185, 19.3961) (19.235, 19.4206) (19.2563, 19.4524) (19.2805, 19.4893) (19.3045, 19.5263) (19.3281, 19.5636) (19.3516, 19.6011) (19.3747, 19.6388) (19.3976, 19.6767) (19.4203, 19.7148) (19.4428, 19.7532) (19.465, 19.7917) (19.487, 19.8303) (19.5088, 19.8692) (19.5304, 19.9082) (19.5518, 19.9474) (19.573, 19.9868) (19.5939, 20.0263) (19.6147, 20.066) (19.6353, 20.1058) (19.6557, 20.1458) (19.6758, 20.186) (19.6958, 20.2263) (19.7157, 20.2667) (19.7353, 20.3073) (19.7547, 20.348) (19.774, 20.3889) (19.7931, 20.4299) (19.812, 20.471) (19.8307, 20.5123) (19.8493, 20.5537) (19.8677, 20.5952) (19.8859, 20.6369) (19.9039, 20.6787) (19.9218, 20.7206) (19.9395, 20.7626) (19.957, 20.8048) (19.9744, 20.847) (19.9916, 20.8894) (20.0087, 20.9319) (20.0255, 20.9746) (20.0423, 21.0173) (20.0588, 21.0602) (20.0752, 21.1031) (20.0915, 21.1462) (20.1075, 21.1894) (20.1235, 21.2327) (20.1392, 21.2761) (20.1548, 21.3196) (20.1703, 21.3632) (20.1856, 21.4069) (20.2008, 21.4507) (20.2158, 21.4946) (20.2306, 21.5387) (20.2453, 21.5828) (20.2598, 21.627) (20.2742, 21.6713) (20.2885, 21.7157) (20.3026, 21.7602) (20.3137, 21.7959) (20.3221, 21.8227) (20.3276, 21.8406) (20.3303, 21.8495) knots 0.13777296 0.13777296 0.13777296 0.13777296 0.13777296 0.13777296 0.14285714 0.15714286 0.17142857 0.18571429 0.2 0.21428571 0.22857143 0.24285714 0.25714286 0.27142857 0.28571429 0.3 0.31428571 0.32857143 0.34285714 0.35714286 0.37142857 0.38571429 0.4 0.41428571 0.42857143 0.44285714 0.45714286 0.47142857 0.48571429 0.5 0.51428571 0.52857143 0.54285714 0.55714286 0.57142857 0.58571429 0.6 0.61428571 0.62857143 0.64285714 0.65714286 0.67142857 0.68571429 0.7 0.71428571 0.72857143 0.74285714 0.75714286 0.77142857 0.78571429 0.8 0.81428571 0.82857143 0.84285714 0.85714286 0.87142857 0.88571429 0.9 0.91428571 0.92857143 0.94285714 0.95714286 0.97142857 0.98571429 1 1 1 1 1 1
  arc A13 (20.3303, 21.8495) -> (19.6048, 22.5028) centre (0, 0) ccw
  spline S26 degree 5 poles (19.6048, 22.5028) (19.5961, 22.4992) (19.5789, 22.4918) (19.5531, 22.4808) (19.5188, 22.4659) (19.476, 22.4473) (19.4334, 22.4284) (19.3908, 22.4095) (19.3483, 22.3904) (19.306, 22.3712) (19.2638, 22.3518) (19.2217, 22.3323) (19.1797, 22.3127) (19.1378, 22.2929) (19.096, 22.2729) (19.0544, 22.2529) (19.0129, 22.2326) (18.9715, 22.2123) (18.9302, 22.1918) (18.8891, 22.1711) (18.8481, 22.1503) (18.8072, 22.1294) (18.7664, 22.1083) (18.7258, 22.087) (18.6853, 22.0656) (18.645, 22.0441) (18.6047, 22.0224) (18.5646, 22.0005) (18.5247, 21.9785) (18.4849, 21.9564) (18.4452, 21.9341) (18.4057, 21.9116) (18.3663, 21.889) (18.3271, 21.8662) (18.288, 21.8433) (18.249, 21.8202) (18.2102, 21.7969) (18.1716, 21.7735) (18.1331, 21.7499) (18.0948, 21.7261) (18.0567, 21.7022) (18.0187, 21.6781) (17.9809, 21.6538) (17.9432, 21.6293) (17.9058, 21.6047) (17.8685, 21.5799) (17.8313, 21.5549) (17.7944, 21.5297) (17.7577, 21.5044) (17.7211, 21.4788) (17.6847, 21.4531) (17.6486, 21.4271) (17.6126, 21.401) (17.5769, 21.3747) (17.5413, 21.3481) (17.506, 21.3214) (17.4709, 21.2944) (17.4361, 21.2672) (17.4015, 21.2398) (17.3671, 21.2121) (17.333, 21.1842) (17.3036, 21.1597) (17.281, 21.1406) (17.2652, 21.1272) (17.2562, 21.1195) (17.2538, 21.1174) knots -1 -1 -1 -1 -1 -1 -0.98571429 -0.97142857 -0.95714286 -0.94285714 -0.92857143 -0.91428571 -0.9 -0.88571429 -0.87142857 -0.85714286 -0.84285714 -0.82857143 -0.81428571 -0.8 -0.78571429 -0.77142857 -0.75714286 -0.74285714 -0.72857143 -0.71428571 -0.7 -0.68571429 -0.67142857 -0.65714286 -0.64285714 -0.62857143 -0.61428571 -0.6 -0.58571429 -0.57142857 -0.55714286 -0.54285714 -0.52857143 -0.51428571 -0.5 -0.48571429 -0.47142857 -0.45714286 -0.44285714 -0.42857143 -0.41428571 -0.4 -0.38571429 -0.37142857 -0.35714286 -0.34285714 -0.32857143 -0.31428571 -0.3 -0.28571429 -0.27142857 -0.25714286 -0.24285714 -0.22857143 -0.21428571 -0.2 -0.18571429 -0.17142857 -0.15714286 -0.14285714 -0.13777296 -0.13777296 -0.13777296 -0.13777296 -0.13777296 -0.13777296
  spline S27 degree 3 poles (16.9981, 21.1134) (17.0184, 21.0971) (17.0417, 21.0849) (17.0916, 21.0701) (17.1178, 21.0676) (17.1639, 21.0723) (17.1837, 21.0774) (17.221, 21.0934) (17.2384, 21.1042) (17.2538, 21.1174) knots 0 0 0 0 0.007813 0.007813 0.015626 0.015626 0.021719 0.021719 0.027811 0.027811 0.027811 0.027811
  arc A14 (16.9981, 21.1134) -> (16.3741, 21.601) centre (0, 0) ccw
  spline S28 degree 3 poles (16.3161, 21.8501) (16.3044, 21.8268) (16.2974, 21.8014) (16.2935, 21.7495) (16.2966, 21.7234) (16.3109, 21.6793) (16.3201, 21.6611) (16.3436, 21.628) (16.3579, 21.6133) (16.3741, 21.601) knots 0 0 0 0 0.007813 0.007813 0.015626 0.015626 0.021719 0.021719 0.027811 0.027811 0.027811 0.027811
  spline S29 degree 5 poles (16.3161, 21.8501) (16.3175, 21.8529) (16.3228, 21.8635) (16.332, 21.8821) (16.345, 21.9086) (16.3617, 21.9431) (16.3805, 21.9829) (16.3991, 22.0229) (16.4173, 22.0631) (16.4353, 22.1035) (16.453, 22.1441) (16.4704, 22.1848) (16.4875, 22.2258) (16.5044, 22.2668) (16.5211, 22.308) (16.5375, 22.3494) (16.5537, 22.3909) (16.5696, 22.4326) (16.5854, 22.4744) (16.6008, 22.5163) (16.6161, 22.5583) (16.6312, 22.6005) (16.646, 22.6429) (16.6606, 22.6853) (16.675, 22.7279) (16.6892, 22.7706) (16.7032, 22.8134) (16.717, 22.8563) (16.7306, 22.8993) (16.744, 22.9425) (16.7572, 22.9857) (16.7702, 23.0291) (16.783, 23.0726) (16.7956, 23.1162) (16.808, 23.1598) (16.8202, 23.2036) (16.8323, 23.2475) (16.8442, 23.2915) (16.8558, 23.3356) (16.8673, 23.3798) (16.8787, 23.4241) (16.8898, 23.4684) (16.9008, 23.5129) (16.9115, 23.5575) (16.9222, 23.6021) (16.9326, 23.6469) (16.9429, 23.6917) (16.9529, 23.7366) (16.9629, 23.7816) (16.9726, 23.8267) (16.9822, 23.8719) (16.9916, 23.9171) (17.0008, 23.9624) (17.0099, 24.0079) (17.0188, 24.0534) (17.0275, 24.0989) (17.0361, 24.1446) (17.0445, 24.1903) (17.0528, 24.2361) (17.0609, 24.282) (17.0688, 24.328) (17.0766, 24.374) (17.0827, 24.4109) (17.0871, 24.4386) (17.0901, 24.4571) (17.0916, 24.4663) knots 0.13777296 0.13777296 0.13777296 0.13777296 0.13777296 0.13777296 0.14285714 0.15714286 0.17142857 0.18571429 0.2 0.21428571 0.22857143 0.24285714 0.25714286 0.27142857 0.28571429 0.3 0.31428571 0.32857143 0.34285714 0.35714286 0.37142857 0.38571429 0.4 0.41428571 0.42857143 0.44285714 0.45714286 0.47142857 0.48571429 0.5 0.51428571 0.52857143 0.54285714 0.55714286 0.57142857 0.58571429 0.6 0.61428571 0.62857143 0.64285714 0.65714286 0.67142857 0.68571429 0.7 0.71428571 0.72857143 0.74285714 0.75714286 0.77142857 0.78571429 0.8 0.81428571 0.82857143 0.84285714 0.85714286 0.87142857 0.88571429 0.9 0.91428571 0.92857143 0.94285714 0.95714286 0.97142857 0.98571429 1 1 1 1 1 1
  arc A15 (17.0916, 24.4663) -> (16.2822, 25.0123) centre (0, 0) ccw
  spline S30 degree 5 poles (16.2822, 25.0123) (16.2742, 25.0075) (16.2581, 24.9978) (16.2341, 24.9833) (16.2022, 24.9638) (16.1624, 24.9393) (16.1228, 24.9148) (16.0833, 24.8901) (16.0439, 24.8653) (16.0046, 24.8403) (15.9655, 24.8153) (15.9265, 24.7901) (15.8877, 24.7648) (15.849, 24.7394) (15.8104, 24.7138) (15.772, 24.6882) (15.7337, 24.6624) (15.6955, 24.6364) (15.6575, 24.6104) (15.6196, 24.5842) (15.5819, 24.5579) (15.5443, 24.5315) (15.5069, 24.5049) (15.4696, 24.4782) (15.4325, 24.4514) (15.3956, 24.4244) (15.3587, 24.3974) (15.3221, 24.3701) (15.2856, 24.3428) (15.2492, 24.3153) (15.2131, 24.2877) (15.177, 24.2599) (15.1412, 24.2321) (15.1055, 24.204) (15.07, 24.1759) (15.0346, 24.1476) (14.9995, 24.1191) (14.9645, 24.0906) (14.9297, 24.0618) (14.895, 24.033) (14.8606, 24.004) (14.8263, 23.9748) (14.7923, 23.9455) (14.7584, 23.9161) (14.7247, 23.8865) (14.6912, 23.8567) (14.6579, 23.8268) (14.6249, 23.7967) (14.592, 23.7665) (14.5594, 23.7361) (14.527, 23.7055) (14.4947, 23.6748) (14.4628, 23.6439) (14.431, 23.6129) (14.3995, 23.5817) (14.3683, 23.5503) (14.3373, 23.5187) (14.3066, 23.4869) (14.2761, 23.4549) (14.246, 23.4227) (14.2161, 23.3903) (14.1903, 23.3619) (14.1706, 23.34) (14.1569, 23.3245) (14.149, 23.3155) (14.1469, 23.3132) knots -1 -1 -1 -1 -1 -1 -0.98571429 -0.97142857 -0.95714286 -0.94285714 -0.92857143 -0.91428571 -0.9 -0.88571429 -0.87142857 -0.85714286 -0.84285714 -0.82857143 -0.81428571 -0.8 -0.78571429 -0.77142857 -0.75714286 -0.74285714 -0.72857143 -0.71428571 -0.7 -0.68571429 -0.67142857 -0.65714286 -0.64285714 -0.62857143 -0.61428571 -0.6 -0.58571429 -0.57142857 -0.55714286 -0.54285714 -0.52857143 -0.51428571 -0.5 -0.48571429 -0.47142857 -0.45714286 -0.44285714 -0.42857143 -0.41428571 -0.4 -0.38571429 -0.37142857 -0.35714286 -0.34285714 -0.32857143 -0.31428571 -0.3 -0.28571429 -0.27142857 -0.25714286 -0.24285714 -0.22857143 -0.21428571 -0.2 -0.18571429 -0.17142857 -0.15714286 -0.14285714 -0.13777296 -0.13777296 -0.13777296 -0.13777296 -0.13777296 -0.13777296
  spline S31 degree 3 poles (13.8943, 23.2736) (13.9167, 23.2603) (13.9414, 23.2514) (13.9929, 23.2437) (14.0192, 23.2449) (14.0642, 23.256) (14.0831, 23.2638) (14.1178, 23.2848) (14.1335, 23.2979) (14.1469, 23.3132) knots 0 0 0 0 0.007813 0.007813 0.015626 0.015626 0.021719 0.021719 0.027811 0.027811 0.027811 0.027811
  arc A16 (13.8943, 23.2736) -> (13.2084, 23.6696) centre (0, 0) ccw
  spline S32 degree 3 poles (13.1164, 23.9082) (13.108, 23.8835) (13.1046, 23.8574) (13.108, 23.8055) (13.1147, 23.78) (13.135, 23.7384) (13.1466, 23.7216) (13.1746, 23.6921) (13.1907, 23.6795) (13.2084, 23.6696) knots 0 0 0 0 0.007813 0.007813 0.015626 0.015626 0.021719 0.021719 0.027811 0.027811 0.027811 0.027811
  spline S33 degree 5 poles (13.1164, 23.9082) (13.1174, 23.9111) (13.1211, 23.9224) (13.1277, 23.9421) (13.1369, 23.9701) (13.1486, 24.0067) (13.1617, 24.0487) (13.1745, 24.0909) (13.187, 24.1333) (13.1991, 24.1758) (13.211, 24.2184) (13.2226, 24.2612) (13.2339, 24.3041) (13.2449, 24.3471) (13.2556, 24.3902) (13.2661, 24.4335) (13.2764, 24.4768) (13.2864, 24.5203) (13.2961, 24.5639) (13.3056, 24.6075) (13.3149, 24.6513) (13.3239, 24.6952) (13.3327, 24.7392) (13.3413, 24.7832) (13.3496, 24.8274) (13.3577, 24.8716) (13.3656, 24.916) (13.3733, 24.9604) (13.3808, 25.0049) (13.3881, 25.0495) (13.3951, 25.0942) (13.4019, 25.1389) (13.4086, 25.1838) (13.415, 25.2287) (13.4212, 25.2737) (13.4272, 25.3187) (13.4331, 25.3639) (13.4387, 25.4091) (13.4441, 25.4544) (13.4494, 25.4997) (13.4544, 25.5452) (13.4593, 25.5907) (13.4639, 25.6362) (13.4684, 25.6818) (13.4727, 25.7275) (13.4768, 25.7733) (13.4807, 25.8191) (13.4845, 25.865) (13.488, 25.9109) (13.4914, 25.9569) (13.4946, 26.003) (13.4976, 26.0491) (13.5004, 26.0953) (13.5031, 26.1415) (13.5056, 26.1878) (13.5079, 26.2342) (13.51, 26.2806) (13.512, 26.3271) (13.5138, 26.3736) (13.5154, 26.4201) (13.5169, 26.4668) (13.5182, 26.5134) (13.5191, 26.5508) (13.5197, 26.5789) (13.52, 26.5976) (13.5202, 26.6069) knots 0.13777296 0.13777296 0.13777296 0.13777296 0.13777296 0.13777296 0.14285714 0.15714286 0.17142857 0.18571429 0.2 0.21428571 0.22857143 0.24285714 0.25714286 0.27142857 0.28571429 0.3 0.31428571 0.32857143 0.34285714 0.35714286 0.37142857 0.38571429 0.4 0.41428571 0.42857143 0.44285714 0.45714286 0.47142857 0.48571429 0.5 0.51428571 0.52857143 0.54285714 0.55714286 0.57142857 0.58571429 0.6 0.61428571 0.62857143 0.64285714 0.65714286 0.67142857 0.68571429 0.7 0.71428571 0.72857143 0.74285714 0.75714286 0.77142857 0.78571429 0.8 0.81428571 0.82857143 0.84285714 0.85714286 0.87142857 0.88571429 0.9 0.91428571 0.92857143 0.94285714 0.95714286 0.97142857 0.98571429 1 1 1 1 1 1
  arc A17 (13.5202, 26.6069) -> (12.6427, 27.0349) centre (0, 0) ccw
  spline S34 degree 5 poles (12.6427, 27.0349) (12.6354, 27.029) (12.6209, 27.0172) (12.5991, 26.9995) (12.5702, 26.9758) (12.5343, 26.946) (12.4984, 26.9162) (12.4627, 26.8862) (12.4272, 26.8562) (12.3918, 26.826) (12.3565, 26.7958) (12.3214, 26.7654) (12.2865, 26.7349) (12.2517, 26.7044) (12.217, 26.6737) (12.1825, 26.6429) (12.1482, 26.612) (12.114, 26.5811) (12.08, 26.55) (12.0462, 26.5188) (12.0125, 26.4875) (11.979, 26.4561) (11.9456, 26.4246) (11.9124, 26.3929) (11.8794, 26.3612) (11.8465, 26.3294) (11.8138, 26.2974) (11.7813, 26.2654) (11.749, 26.2332) (11.7168, 26.201) (11.6848, 26.1686) (11.653, 26.1361) (11.6214, 26.1035) (11.5899, 26.0708) (11.5587, 26.0379) (11.5276, 26.005) (11.4968, 25.9719) (11.4661, 25.9388) (11.4356, 25.9055) (11.4053, 25.8721) (11.3753, 25.8386) (11.3454, 25.8049) (11.3157, 25.7712) (11.2863, 25.7373) (11.2571, 25.7033) (11.228, 25.6691) (11.1992, 25.6349) (11.1707, 25.6005) (11.1424, 25.566) (11.1143, 25.5314) (11.0864, 25.4966) (11.0588, 25.4617) (11.0314, 25.4267) (11.0043, 25.3915) (10.9774, 25.3562) (10.9509, 25.3207) (10.9246, 25.2851) (10.8986, 25.2494) (10.8729, 25.2135) (10.8475, 25.1774) (10.8224, 25.1412) (10.8009, 25.1095) (10.7844, 25.085) (10.7729, 25.0677) (10.7664, 25.0578) (10.7647, 25.0552) knots -1 -1 -1 -1 -1 -1 -0.98571429 -0.97142857 -0.95714286 -0.94285714 -0.92857143 -0.91428571 -0.9 -0.88571429 -0.87142857 -0.85714286 -0.84285714 -0.82857143 -0.81428571 -0.8 -0.78571429 -0.77142857 -0.75714286 -0.74285714 -0.72857143 -0.71428571 -0.7 -0.68571429 -0.67142857 -0.65714286 -0.64285714 -0.62857143 -0.61428571 -0.6 -0.58571429 -0.57142857 -0.55714286 -0.54285714 -0.52857143 -0.51428571 -0.5 -0.48571429 -0.47142857 -0.45714286 -0.44285714 -0.42857143 -0.41428571 -0.4 -0.38571429 -0.37142857 -0.35714286 -0.34285714 -0.32857143 -0.31428571 -0.3 -0.28571429 -0.27142857 -0.25714286 -0.24285714 -0.22857143 -0.21428571 -0.2 -0.18571429 -0.17142857 -0.15714286 -0.14285714 -0.13777296 -0.13777296 -0.13777296 -0.13777296 -0.13777296 -0.13777296
  spline S35 degree 3 poles (10.52, 24.9809) (10.544, 24.9708) (10.5698, 24.9654) (10.6218, 24.965) (10.6477, 24.9698) (10.6907, 24.987) (10.7083, 24.9974) (10.7398, 25.023) (10.7535, 25.0382) (10.7647, 25.0552) knots 0 0 0 0 0.007813 0.007813 0.015626 0.015626 0.021719 0.021719 0.027811 0.027811 0.027811 0.027811
  arc A18 (10.52, 24.9809) -> (9.7857, 25.2775) centre (0, 0) ccw
  spline S36 degree 3 poles (9.6613, 25.5009) (9.6565, 25.4753) (9.6568, 25.4491) (9.6673, 25.3981) (9.6775, 25.3738) (9.7034, 25.3354) (9.7173, 25.3204) (9.749, 25.2951) (9.7668, 25.2849) (9.7857, 25.2775) knots 0 0 0 0 0.007813 0.007813 0.015626 0.015626 0.021719 0.021719 0.027811 0.027811 0.027811 0.027811